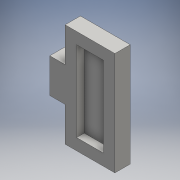
# Autodesk Inventor part: basebaquela
Saved by Autodesk Inventor 2016 (Build 200138000, 138)
## iProperties
Created: 2017-03-25
Part Number: basebaquela
Material: Generic
Document SubType Name: Sheet Metal
Designer: jorge
Density: 1 g/cm^3
Sheet Metal Rule: Default_mm
Appearance: Default
Author: jorge
## iProperties of the stored document basebaquela_3DPrint.ipt
Created: 2017-03-25
Part Number: basebaquela_3DPrint
Material: Generic
Document SubType Name: Modeling
Designer: jorge
Density: 1 g/cm^3
Appearance: Default
Author: jorge
Autodesk Inventor part; units mm, degrees
ref_plane "YZ Plane" through (0, 0, 0) normal (1, 0, 0) x (0, 1, 0)
ref_plane "XZ Plane" through (0, 0, 0) normal (0, 1, 0) x (-1, 0, 0)
ref_plane "XY Plane" through (0, 0, 0) normal (0, 0, 1) x (1, 0, 0)
sketch "Sketch3" plane through (0, 0, 0) normal (0, 1, 0) x (-1, 0, 0)
  line L0 (0, 0) -> (7, 0)
  line L1 (7, 0) -> (7, -21)
  line L2 (7, -21) -> (0, -21)
  line L3 (0, -21) -> (0, 0)
  line L4 (10, -24) -> (10, 3)
  line L5 (10, 3) -> (-3, 3)
  line L6 (-3, 3) -> (-3, -24)
  line L7 (-3, -24) -> (10, -24)
  line L8 (10, -10.5) -> (10, -6)
  line L9 (10, -6) -> (14, -6)
  line L10 (14, -6) -> (14, -15)
  line L11 (14, -15) -> (10, -15)
  dimension "d13" = 7
  dimension "d14" = 21
  dimension "d15" = 3
  dimension "d16" = 4.5
  dimension "d17" = 4
  dimension "d18" = 9
  constraints: 24 end point, 8 perpendicular, 2 point on line, 1 horizontal, 1 midpoint, 1 vertical, 3 other
  measures "d13" distance of L0.start L0.end
  measures "d14" distance of L0.end L1.end
  measures "d15" distance between parallel lines of L1 L4
  measures "d16" distance of L8.start L8.end
  measures "d17" distance of L8.end L9.end
  measures "d18" distance of L9.end L10.end
extrude "Extrusion3" add sketch "Sketch3" along normal blind 2
sketch "Sketch4" plane through (0, 2, 0) normal (0, 1, 0) x (1, 0, 0)
  line L0 (-7, 0) -> (-7, 21) projected
  line L1 (-7, 21) -> (0, 21) projected
  line L2 (0, 21) -> (0, 0) projected
  line L3 (0, 0) -> (-7, 0) projected
  line L4 (-10, 15) -> (-14, 15) projected
  line L5 (-14, 15) -> (-14, 6) projected
  line L6 (-14, 6) -> (-10, 6) projected
  line L7 (-10, 6) -> (-10, -3) projected
  line L8 (-10, -3) -> (3, -3) projected
  line L9 (3, -3) -> (3, 24) projected
  line L10 (3, 24) -> (-10, 24) projected
  line L11 (-10, 24) -> (-10, 15) projected
extrude "Extrusion4" add sketch "Sketch4" along normal blind 2 contours L0 L1 L2 L3 | L11 L10 L9 L8 L7 L6 L5 L4
equation "\"BendRadius\" = Thickness"
equation "\"BendReliefWidth\" = Thickness"
equation "\"BendReliefDepth\" = 0.5 * Thickness"
equation "\"CornerReliefSize\" = 4 * Thickness"
equation "\"MinimumRemnant\" = 2 * Thickness"
equation "\"TransitionRadius\" = BendRadius"
equation "\"JacobiRadiusSize\" = BendRadius"
equation "\"GapSize\" = Thickness"
equation "\"Thickness\" = 0.5"
body "Solid2"
